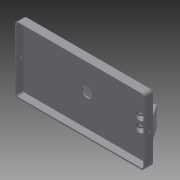
# Autodesk Inventor part: Slave Tablet Enclosure
Saved by Autodesk Inventor 2014 SP2 (Build 180246200, 246)
## iProperties
Created: 2015-08-04
Part Number: Slave Tablet Enclosure
Material: Generic
Document SubType Name: Modeling
Designer: Devon
Density: 1 g/cm^3
Appearance: Default
Author: Devon
Autodesk Inventor part; units mm, degrees
ref_plane "YZ Plane" through (0, 0, 0) normal (1, 0, 0) x (0, 1, 0)
ref_plane "XZ Plane" through (0, 0, 0) normal (0, 1, 0) x (-1, 0, 0)
ref_plane "XY Plane" through (0, 0, 0) normal (0, 0, 1) x (1, 0, 0)
sketch "Sketch1" plane through (0, 0, 0) normal (0, 0, 1) x (1, 0, 0)
  line L0 (-10.4542, 14.6019) -> (210.2083, 14.6019)
  line L1 (216.5583, 8.2519) -> (216.5583, -98.1106)
  line L2 (210.2083, -104.4606) -> (-10.4542, -104.4606)
  line L3 (-16.8042, -98.1106) -> (-16.8042, 8.2519)
  line L4 (99.877, 12.2207) -> (-10.4542, 12.2207)
  line L5 (-14.423, 8.2519) -> (-14.423, -44.9293)
  line L6 (99.877, 12.2207) -> (210.2083, 12.2207)
  line L7 (214.177, 8.2519) -> (214.177, -44.9293)
  line L8 (99.877, -102.0793) -> (210.2083, -102.0793)
  line L9 (214.177, -98.1106) -> (214.177, -44.9293)
  line L10 (99.877, -102.0793) -> (-10.4542, -102.0793)
  line L11 (-14.423, -98.1106) -> (-14.423, -44.9293)
  arc A0 (-10.4542, 14.6019) -> (-16.8042, 8.2519) centre (-10.4542, 8.2519) ccw
  arc A1 (216.5583, 8.2519) -> (210.2083, 14.6019) centre (210.2083, 8.2519) ccw
  arc A2 (210.2083, -104.4606) -> (216.5583, -98.1106) centre (210.2083, -98.1106) ccw
  arc A3 (-16.8042, -98.1106) -> (-10.4542, -104.4606) centre (-10.4542, -98.1106) ccw
  arc A4 (-10.4542, 12.2207) -> (-14.423, 8.2519) centre (-10.4542, 8.2519) ccw
  arc A5 (214.177, 8.2519) -> (210.2083, 12.2207) centre (210.2083, 8.2519) ccw
  arc A6 (210.2083, -102.0793) -> (214.177, -98.1106) centre (210.2083, -98.1106) ccw
  arc A7 (-14.423, -98.1106) -> (-10.4542, -102.0793) centre (-10.4542, -98.1106) ccw
  point P0 (0, 0)
  point P1 (-16.8042, 14.6019)
  point P2 (216.5583, -104.4606)
  point P3 (216.5583, 14.6019)
  point P4 (-16.8042, -104.4606)
  dimension "d0" = 233.3625
  dimension "d1" = 119.0625
  dimension "d9" = 6.35
  dimension "d10" = 3.9688
  constraints: 24 end point, 16 point on circle, 16 tangent, 8 centre point, 8 point on line, 6 equal radius, 4 horizontal, 4 perpendicular, 2 parallel
  measures "d0" distance of point (216.558, -104.461) point (-16.804, -104.461)
  measures "d1" distance of point (216.558, 14.602) point (216.558, -104.461)
  measures "d9" radius of A0
  measures "d10" radius of A4
extrude "Extrusion1" add sketch "Sketch1" along normal blind 2.3813 contours L0 A1 L1 A2 L2 A3 L3 A0 | L6 A5 L7 L9 A6 L8 L10 A7 L11 L5 A4 L4
sketch "Sketch2" plane through (0, 0, 2.3813) normal (0, 0, 1) x (1, 0, 0)
  line L0 (210.2083, 14.6019) -> (-10.4542, 14.6019) projected
  arc A0 (-10.4542, 14.6019) -> (-16.8042, 8.2519) centre (-10.4542, 8.2519) ccw projected
  line L1 (-16.8042, 8.2519) -> (-16.8042, -98.1106) projected
  arc A1 (-16.8042, -98.1106) -> (-10.4542, -104.4606) centre (-10.4542, -98.1106) ccw projected
  line L2 (-10.4542, -104.4606) -> (210.2083, -104.4606) projected
  arc A2 (210.2083, -104.4606) -> (216.5583, -98.1106) centre (210.2083, -98.1106) ccw projected
  line L3 (216.5583, -98.1106) -> (216.5583, 8.2519) projected
  arc A3 (216.5583, 8.2519) -> (210.2083, 14.6019) centre (210.2083, 8.2519) ccw projected
  line L4 (99.877, 12.2207) -> (-10.4542, 12.2207)
  line L5 (-14.423, 8.2519) -> (-14.423, -44.9293)
  line L6 (99.877, -102.0793) -> (-10.4542, -102.0793)
  line L7 (-14.423, -98.1106) -> (-14.423, -44.9293)
  line L8 (99.877, -102.0793) -> (210.2083, -102.0793)
  line L9 (214.177, -98.1106) -> (214.177, -44.9293)
  line L10 (99.877, 12.2207) -> (210.2083, 12.2207)
  line L11 (214.177, 8.2519) -> (214.177, -44.9293)
  arc A4 (-10.4542, 12.2207) -> (-14.423, 8.2519) centre (-10.4542, 8.2519) ccw
  arc A5 (214.177, 8.2519) -> (210.2083, 12.2207) centre (210.2083, 8.2519) ccw
  arc A6 (210.2083, -102.0793) -> (214.177, -98.1106) centre (210.2083, -98.1106) ccw
  arc A7 (-14.423, -98.1106) -> (-10.4542, -102.0793) centre (-10.4542, -98.1106) ccw
  point P0 (0, 0)
  dimension "d15" = 3.9688
  constraints: 16 end point, 8 point on circle, 8 tangent, 4 centre point, 3 equal radius, 2 horizontal, 2 perpendicular
  measures "d15" radius of A4
extrude "Extrusion2" add sketch "Sketch2" along normal blind 2.3813
sketch "Sketch3" plane through (0, 0, 4.7625) normal (0, 0, 1) x (1, 0, 0)
  arc A0 (-10.4542, 12.2207) -> (-14.423, 8.2519) centre (-10.4542, 8.2519) ccw projected
  line L0 (-10.4542, 12.2207) -> (210.2083, 12.2207) projected
  arc A1 (214.177, 8.2519) -> (210.2083, 12.2207) centre (210.2083, 8.2519) ccw projected
  line L1 (214.177, 8.2519) -> (214.177, -98.1106) projected
  arc A2 (210.2083, -102.0793) -> (214.177, -98.1106) centre (210.2083, -98.1106) ccw projected
  line L2 (210.2083, -102.0793) -> (-10.4542, -102.0793) projected
  arc A3 (-14.423, -98.1106) -> (-10.4542, -102.0793) centre (-10.4542, -98.1106) ccw projected
  line L3 (-14.423, -98.1106) -> (-14.423, 8.2519) projected
  line L4 (210.2083, 14.6019) -> (-10.4542, 14.6019) projected
  arc A4 (-10.4542, 14.6019) -> (-16.8042, 8.2519) centre (-10.4542, 8.2519) ccw projected
  line L5 (-16.8042, 8.2519) -> (-16.8042, -98.1106) projected
  arc A5 (-16.8042, -98.1106) -> (-10.4542, -104.4606) centre (-10.4542, -98.1106) ccw projected
  line L6 (-10.4542, -104.4606) -> (210.2083, -104.4606) projected
  arc A6 (210.2083, -104.4606) -> (216.5583, -98.1106) centre (210.2083, -98.1106) ccw projected
  line L7 (216.5583, -98.1106) -> (216.5583, 8.2519) projected
  arc A7 (216.5583, 8.2519) -> (210.2083, 14.6019) centre (210.2083, 8.2519) ccw projected
  line L8 (214.177, -44.9293) -> (214.177, -41.7543)
  line L9 (214.177, -41.7543) -> (216.5583, -41.7543)
  line L10 (216.5583, -41.7543) -> (216.5583, -44.9293)
  line L11 (216.5583, -44.9293) -> (216.5583, -48.1043)
  line L12 (216.5583, -48.1043) -> (214.177, -48.1043)
  line L13 (214.177, -48.1043) -> (214.177, -44.9293)
  line L14 (-14.423, -44.9293) -> (-14.423, -41.7543)
  line L15 (-14.423, -41.7543) -> (-16.8042, -41.7543)
  line L16 (-16.8042, -41.7543) -> (-16.8042, -44.9293)
  line L17 (-16.8042, -44.9293) -> (-16.8042, -48.1043)
  line L18 (-16.8042, -48.1043) -> (-14.423, -48.1043)
  line L19 (-14.423, -48.1043) -> (-14.423, -44.9293)
  point P0 (0, 0)
  dimension "d18" = 3.175
  dimension "d19" = 3.175
  dimension "d20" = 3.175
  dimension "d21" = 3.175
  constraints: 24 end point, 8 point on line, 4 midpoint, 4 perpendicular, 3 collinear
  measures "d18" distance of L8.start L8.end
  measures "d19" distance of L9.end L10.end
  measures "d20" distance of L10.end L11.end
  measures "d21" distance of L14.start L14.end
extrude "Extrusion3" add sketch "Sketch3" along normal blind 10.3188 contours A0 L3 L15 L5 A4 L4 A7 L7 L9 L1 A1 L0 | L3 A3 L2 A2 L1 L12 L7 A6 L6 A5 L5 L18
sketch "Sketch4" plane through (0, 0, 15.0813) normal (0, 0, 1) x (1, 0, 0)
  line L0 (214.177, -41.7543) -> (216.5583, -41.7543)
  line L1 (216.5583, -41.7543) -> (216.5583, -48.1043)
  line L2 (216.5583, -48.1043) -> (214.177, -48.1043)
  line L3 (214.177, -48.1043) -> (214.177, -41.7543)
  line L4 (-16.8042, -41.7543) -> (-14.423, -41.7543)
  line L5 (-14.423, -41.7543) -> (-14.423, -48.1043)
  line L6 (-14.423, -48.1043) -> (-16.8042, -48.1043)
  line L7 (-16.8042, -48.1043) -> (-16.8042, -41.7543)
  point P0 (0, 0)
  dimension "d24" = 2.3813
  dimension "d25" = 6.35
  dimension "d26" = 2.3813
  dimension "d27" = 6.35
  constraints: 16 end point, 4 parallel, 2 horizontal, 2 perpendicular
  measures "d24" distance of L1.end L2.end
  measures "d25" distance of L0.end L1.end
  measures "d26" distance of L5.end L6.end
  measures "d27" distance of L4.end L5.end
extrude "Extrusion4" add sketch "Sketch4" against normal blind 7.9375
sketch "Sketch5" plane through (0, 0, 0) normal (0, 0, -1) x (-1, 0, 0)
  arc A0 (-210.2083, 14.6019) -> (-216.5583, 8.2519) centre (-210.2083, 8.2519) ccw projected
  line L0 (-210.2083, 8.2519) -> (-99.877, 8.2519)
  line L1 (-99.877, 8.2519) -> (-99.877, -44.9293)
  line L2 (-99.877, -44.9293) -> (-210.2083, -44.9293)
  line L3 (-210.2083, -44.9293) -> (-210.2083, 8.2519)
  point P0 (0, 0)
  constraints: 8 end point, 2 parallel, 1 horizontal, 1 perpendicular
hole "Hole1" at (99.877, -44.9293, 0) direction (0, 0, 1) diameter 19.05 end through all
sketch "Sketch6" plane through (0, 0, 0) normal (0, 0, -1) x (-1, 0, 0)
  line L0 (-216.5583, 8.2519) -> (-216.5583, -98.1106) projected
  line L1 (-216.5583, -25.8793) -> (-216.5583, -63.9793)
  line L2 (-216.5583, -63.9793) -> (-170.0509, -63.9793)
  line L3 (-170.0509, -63.9793) -> (-170.0509, -25.8793)
  line L4 (-170.0509, -25.8793) -> (-216.5583, -25.8793)
  point P0 (0, 0)
  dimension "d39" = 38.1
  dimension "d43" = 46.5074
  constraints: 8 end point, 2 perpendicular, 2 point on line, 1 parallel
  measures "d39" distance of L1.end L1.start
  measures "d43" distance of L1.end L2.end
extrude "Extrusion6" add sketch "Sketch6" along normal blind 38.1
sketch "Sketch8" plane through (170.0509, -25.8793, 0) normal (0, 1, 0) x (1, 0, 0)
  line L0 (46.5074, 0) -> (13.7658, 46.7599)
  point P0 (46.5074, 38.1)
  point P1 (0, 38.1)
  point P2 (-170.0509, 0)
  constraints: 2 end point
split body "Split1" sketch "Sketch8" result one side removed curves L0 removed pieces at (208.0752, -38.5793, -12.9868)
sketch "Sketch9" plane through (170.0509, -25.8793, 0) normal (0, 1, 0) x (1, 0, 0)
  line L0 (0, 0) -> (64.0379, 44.8398)
  line L1 (0, 0) -> (78.1758, 0) construction
  line L2 (0, 0) -> (0, 38.1)
  point P0 (-170.0509, 0)
  dimension "d48" = 35
  constraints: 6 end point, 1 equal length, 1 horizontal, 1 perpendicular
  measures "d48" angle of L1 L0
split body "Split2" sketch "Sketch9" result one side removed curves L2 L0 removed pieces at (170.5509, -51.2793, -12.7)
ref_plane "Work Plane1" through (204.9, -63.9793, -16.6497) normal (-0.5735764, 0, -0.819152) x (-0.819152, 0, 0.5735764)
sketch "Sketch10" plane through (204.9, -63.9793, -16.6497) normal (-0.5735764, 0, -0.819152) x (-0.819152, 0, 0.5735764)
  line L0 (0, 38.1) -> (38.0966, 38.1) projected
  line L1 (0, 0) -> (0, 38.1) projected
  line L2 (38.0966, 0) -> (0, 0) projected
  line L3 (38.0966, 38.1) -> (38.0966, 0) projected
  line L4 (19.0483, 38.1) -> (19.0483, 28.575)
  line L5 (19.0483, 0) -> (19.0483, 9.525)
  point P0 (177.3942, 63.9793)
  dimension "d50" = 9.525
  dimension "d51" = 9.525
  constraints: 4 end point, 2 midpoint, 1 collinear, 1 parallel
  measures "d50" distance of L4.start L4.end
  measures "d51" distance of L5.start L5.end
hole "Hole2" at (189.2966, -35.4043, -5.724) at (189.2966, -54.4543, -5.724) direction (0.5735764, 0, 0.819152) diameter 13.4938 end through all
sketch "Sketch11" plane through (204.9, -63.9793, -16.6497) normal (-0.5735764, 0, -0.819152) x (-0.819152, 0, 0.5735764)
  line L0 (0, 38.1) -> (38.0966, 38.1) projected
  line L1 (0, 0) -> (0, 38.1) projected
  line L2 (38.0966, 0) -> (0, 0) projected
  line L3 (38.0966, 38.1) -> (38.0966, 0) projected
  line L4 (19.0483, 38.1) -> (19.0483, 28.575)
  line L5 (19.0483, 0) -> (19.0483, 9.525)
  point P0 (177.3942, 63.9793)
  dimension "d59" = 9.525
  dimension "d60" = 9.525
  constraints: 4 end point, 2 midpoint, 1 collinear, 1 parallel
  measures "d59" distance of L4.start L4.end
  measures "d60" distance of L5.start L5.end
hole "Hole3" at (189.2966, -35.4043, -5.724) at (189.2966, -54.4543, -5.724) direction (-0.5735764, 0, -0.819152) diameter 8.3312 end through all
body "Solid1"
